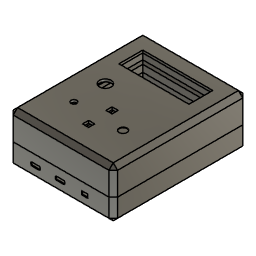
Enclosure (Autodesk Fusion 360 design; units mm, degrees)
Autodesk Fusion 360 part; units mm, degrees
sketch "Sketch1" plane through (0, 0, 0) normal (0, 0, 1) x (1, 0, 0)
  line L0 (0, 0) -> (100, 0)
  line L1 (100, 0) -> (100, -130)
  line L2 (100, -130) -> (0, -130)
  line L3 (0, -130) -> (0, 0)
  line L4 (-3, -133) -> (-3, 3)
  line L5 (-3, 3) -> (103, 3)
  line L6 (103, 3) -> (103, -133)
  line L7 (103, -133) -> (-3, -133)
  dimension "d1" = 100
  dimension "d2" = 130
  dimension "d3" = -3
  constraint horizontal L0
  constraint vertical L1
  constraint horizontal L2
  constraint vertical L3
  constraint coincident L0.start L3.end
  measures "d1" distance of L0.start L0.end
  measures "d2" distance of L0.start L2.end
extrude "Extrude1" add sketch "Sketch1" against normal blind 3 contours L0 L1 L2 L3 | L4 L5 L6 L7 makes body 1
extrude "Extrude2" add sketch "Sketch1" along normal blind 20 separate body makes body 2
extrude "Extrude5" add 1 faces at (-2, -43.3333, 20) along direction (0, 0, 1) blind 25 separate body on bodies 2 makes body 3
sketch "Sketch2" plane through (0, 0, 45) normal (0, 0, 1) x (-1, 0, 0)
  line L0 (-100, 130) -> (0, 130)
  line L1 (0, 130) -> (0, 0)
  line L2 (0, 0) -> (-100, 0)
  line L3 (-100, 0) -> (-100, 130)
  line L4 (-102, 132) -> (-102, -2)
  line L5 (-102, -2) -> (2, -2)
  line L6 (2, -2) -> (2, 132)
  line L7 (2, 132) -> (-102, 132)
  line L8 (2, -2) -> (-102, -2)
  line L9 (-102, -2) -> (-102, 132)
  line L10 (-102, 132) -> (2, 132)
  line L11 (2, 132) -> (2, -2)
  line L12 (0, 0) -> (-100, 0)
  line L13 (-100, 0) -> (-100, 130)
  line L14 (-100, 130) -> (0, 130)
  line L15 (0, 130) -> (0, 0)
  line L16 (0, 0) -> (-14.45, 0)
  line L17 (-14.45, 0) -> (-14.45, 14.45)
  line L18 (-14.45, 14.45) -> (0, 14.45)
  line L19 (0, 14.45) -> (0, 0)
  line L20 (-14.45, 14.45) -> (-85.55, 14.45)
  line L21 (-85.55, 14.45) -> (-85.55, 38.65)
  line L22 (-85.55, 38.65) -> (-14.45, 38.65)
  line L23 (-14.45, 38.65) -> (-14.45, 14.45)
  line L24 (-85.55, 14.45) -> (-100, 14.45)
  circle A0 centre (-25, 95) radius 2.9
  circle A1 centre (-25, 63) radius 5.95
  line L25 (-48.8, 103.8) -> (-55, 103.8)
  line L26 (-55, 103.8) -> (-55, 110)
  line L27 (-55, 110) -> (-48.8, 110)
  line L28 (-48.8, 110) -> (-48.8, 103.8)
  line L29 (-48.8, 80) -> (-55, 80)
  line L30 (-55, 80) -> (-55, 86.2)
  line L31 (-55, 86.2) -> (-48.8, 86.2)
  line L32 (-48.8, 86.2) -> (-48.8, 80)
  circle A2 centre (-75, 95) radius 4
  line L33 (-100, 130) -> (-75, 130)
  line L34 (-75, 130) -> (-75, 95)
  line L35 (-75, 95) -> (-100, 95)
  line L36 (-100, 95) -> (-100, 130)
  line L37 (-55, 110) -> (-100, 110)
  line L38 (-100, 110) -> (-100, 130)
  line L39 (-100, 130) -> (-55, 130)
  line L40 (-55, 130) -> (-55, 110)
  line L41 (-75, 95) -> (-25, 95)
  line L42 (-25, 95) -> (-25, 63)
  line L43 (-25, 63) -> (-25, 65.0002)
  line L44 (-48.8, 86.2) -> (-48.8, 95)
  line L45 (-48.8, 95) -> (-48.8, 103.8)
  line L46 (-100, 130) -> (0, 130)
  line L47 (0, 130) -> (0, 0)
  line L48 (0, 0) -> (-100, 0)
  line L49 (-100, 0) -> (-100, 130)
  line L50 (-103, 133) -> (-103, -3)
  line L51 (-103, -3) -> (3, -3)
  line L52 (3, -3) -> (3, 133)
  line L53 (3, 133) -> (-103, 133)
  dimension "d8" = 71.1
  dimension "d9" = 24.2
  dimension "d11" = 5.8
  dimension "d12" = 11.9
  dimension "d15" = 6.2
  dimension "d16" = 8
  dimension "d17" = 25
  dimension "d19" = 45
  dimension "d20" = 20
  dimension "d22" = 50
  dimension "d23" = 32
  dimension "d27" = 35
  constraint horizontal L8
  constraint vertical L9
  constraint horizontal L10
  constraint vertical L11
  constraint coincident L4.start L7.end
  constraint coincident L5.end L6.start
  constraint horizontal L12
  constraint vertical L13
  constraint horizontal L14
  constraint vertical L15
  constraint coincident L0.start L3.end
  constraint coincident L1.end L2.start
  constraint horizontal L16
  constraint vertical L17
  constraint horizontal L18
  constraint vertical L19
  constraint horizontal L20
  constraint vertical L21
  constraint horizontal L22
  constraint vertical L23
  constraint coincident L13 L24.end
  constraint perpendicular L13 L24
  constraint equal L18 L24
  constraint equal L17 L18
  constraint horizontal L25
  constraint vertical L26
  constraint horizontal L27
  constraint vertical L28
  constraint horizontal L29
  constraint vertical L30
  constraint horizontal L31
  constraint vertical L32
  constraint equal L25 L26
  constraint equal L26 L32
  constraint equal L29 L32
  constraint horizontal L33
  constraint vertical L34
  constraint horizontal L35
  constraint vertical L36
  constraint coincident A2.centre L34.end
  constraint horizontal L37
  constraint vertical L38
  constraint horizontal L39
  constraint vertical L40
  constraint perpendicular L34 L41
  constraint coincident A0.centre L41.end
  constraint perpendicular L41 L42
  constraint coincident A1.centre L42.end
  constraint parallel L42 L43
  constraint coincident L41 L44.end
  constraint perpendicular L41 L44
  constraint perpendicular L25 L45
  constraint equal L44 L45
  measures "d8" distance of L17.end L20.end
  measures "d9" distance of L17.end L22.end
  measures "d11" diameter of A0
  measures "d12" diameter of A1
  measures "d15" distance of L25.start L25.end
  measures "d16" diameter of A2
  measures "d17" distance of A2.centre L35.end
  measures "d19" distance of L26.end L37.end
  measures "d20" distance of L26.end L39.end
  measures "d22" distance of A2.centre A0.centre
  measures "d23" distance of A0.centre A1.centre
  measures "d27" distance of L14 L41
extrude "Extrude3" add sketch "Sketch2" along normal blind 3 separate body contours L0 L3 L13 L14 L33 L34 L36 L37 L38 L39 L46 L49 | L0 L14 L34 L37 L39 L40 L46 | L3 L13 A2 L34 L35 L36 L37 L49 | L0 L1 L3 L13 L14 L15 L18 L21 L22 L23 L24 L27 L28 A2 L35 L40 L41 L45 L46 L47 L49 | L25 L26 A2 L34 L37 L41 L45 | L2 L3 L12 L13 L17 L20 L24 L48 L49 | L1 L2 L12 L15 L16 L17 L18 L19 L47 L48 | L4 L5 L6 L7 L8 L9 L10 L11 | L50 L51 L52 L53 makes body 4
sketch "Sketch6" plane through (0, 0, 45) normal (0, 0, -1) x (1, 0, 0)
  line L0 (48.8, 86.2) -> (55, 86.2)
  line L1 (55, 86.2) -> (55, 80)
  line L2 (55, 80) -> (48.8, 80)
  line L3 (48.8, 80) -> (48.8, 86.2)
  line L4 (14.45, 38.65) -> (85.55, 38.65)
  line L5 (85.55, 38.65) -> (85.55, 14.45)
  line L6 (85.55, 14.45) -> (14.45, 14.45)
  line L7 (14.45, 14.45) -> (14.45, 38.65)
  circle A0 centre (25, 95) radius 2.9
  circle A1 centre (25, 63) radius 5.95
  circle A2 centre (75, 95) radius 4
  line L8 (48.8, 110) -> (55, 110)
  line L9 (55, 110) -> (55, 103.8)
  line L10 (55, 103.8) -> (48.8, 103.8)
  line L11 (48.8, 103.8) -> (48.8, 110)
  line L12 (103, 133) -> (-3, 133)
  line L13 (-3, 133) -> (-3, -3)
  line L14 (-3, -3) -> (103, -3)
  line L15 (103, -3) -> (103, 133)
  line L16 (5, 5) -> (95, 5)
  line L17 (95, 5) -> (95, 125)
  line L18 (95, 125) -> (5, 125)
  line L19 (5, 125) -> (5, 5)
  line L20 (5, 5) -> (95, 125) construction
  line L21 (95, 5) -> (5, 125) construction
  line L22 (46.9, 78.1) -> (56.9, 78.1)
  line L23 (56.9, 78.1) -> (56.9, 88.1)
  line L24 (56.9, 88.1) -> (46.9, 88.1)
  line L25 (46.9, 88.1) -> (46.9, 78.1)
  line L26 (46.9, 78.1) -> (56.9, 88.1) construction
  line L27 (56.9, 78.1) -> (46.9, 88.1) construction
  line L28 (46.9, 101.9) -> (56.9, 101.9)
  line L29 (56.9, 101.9) -> (56.9, 111.9)
  line L30 (56.9, 111.9) -> (46.9, 111.9)
  line L31 (46.9, 111.9) -> (46.9, 101.9)
  line L32 (46.9, 101.9) -> (56.9, 111.9) construction
  line L33 (56.9, 101.9) -> (46.9, 111.9) construction
  circle A3 centre (25, 95) radius 5
  circle A4 centre (25, 63) radius 10
  line L34 (10, 11.55) -> (90, 11.55)
  line L35 (90, 11.55) -> (90, 41.55)
  line L36 (90, 41.55) -> (10, 41.55)
  line L37 (10, 41.55) -> (10, 11.55)
  line L38 (10, 11.55) -> (90, 41.55) construction
  line L39 (90, 11.55) -> (10, 41.55) construction
  point P0 (50, 65)
  point P1 (51.9, 83.1)
  point P2 (51.9, 106.9)
  point P3 (50, 26.55)
  dimension "d68" = 90
  dimension "d69" = 120
  dimension "d70" = 10
  dimension "d71" = 10
  dimension "d72" = 10
  dimension "d73" = 10
  dimension "d74" = 10
  dimension "d75" = 20
  dimension "d76" = 80
  dimension "d77" = 30
  constraint horizontal L16
  constraint perpendicular L16 L17
  constraint parallel L16 L18
  constraint parallel L17 L19
  constraint coincident L20 P0
  constraint coincident L21 P0
  constraint horizontal L22
  constraint perpendicular L22 L23
  constraint parallel L22 L24
  constraint parallel L23 L25
  constraint coincident L26 P1
  constraint coincident L27 P1
  constraint horizontal L28
  constraint perpendicular L28 L29
  constraint parallel L28 L30
  constraint parallel L29 L31
  constraint coincident L32 P2
  constraint coincident L33 P2
  constraint concentric A0 A3
  constraint concentric A1 A4
  constraint horizontal L34
  constraint perpendicular L34 L35
  constraint parallel L34 L36
  constraint parallel L35 L37
  constraint coincident L38 P3
  constraint coincident L39 P3
  measures "d68" distance of L17.end L18.end
  measures "d69" distance of L16.end L17.end
  measures "d70" distance of L23.end L24.end
  measures "d71" distance of L22.end L23.end
  measures "d72" distance of L29.end L30.end
  measures "d73" distance of L28.end L29.end
  measures "d74" diameter of A3
  measures "d75" diameter of A4
  measures "d76" distance of L35.end L36.end
  measures "d77" distance of L34.end L35.end
extrude "Extrude10" cut sketch "Sketch6" against normal blind 2 contours A2 | L16 L17 L18 L19 bodies 4
chamfer "Chamfer1" distance 0.5 angle 45 15 edges at (55, -83.1, 45) (51.9, -86.2, 45) (48.8, -83.1, 45) (51.9, -80, 45) (51.9, -103.8, 45) (55, -106.9, 45) (51.9, -110, 45) (48.8, -106.9, 45) (27.7037, -96.0487, 45) (50, -38.65, 45) (85.55, -26.55, 45) (50, -14.45, 45) (14.45, -26.55, 45) (30.5473, -65.1516, 45) (78.7293, -96.4465, 47) on bodies 4
sketch "Sketch3" plane through (0, -133, 0) normal (0, -1, 0) x (1, 0, 0)
  line L0 (-3, 0) -> (103, 0)
  line L1 (103, 0) -> (103, 20)
  line L2 (103, 20) -> (-3, 20)
  line L3 (-3, 20) -> (-3, 0)
  line L4 (49, 0) -> (49, 10)
  line L5 (49, 10) -> (24, 10)
  line L6 (28.75, 8.25) -> (19.25, 8.25)
  line L7 (19.25, 8.25) -> (19.25, 11.75)
  line L8 (19.25, 11.75) -> (28.75, 11.75)
  line L9 (28.75, 11.75) -> (28.75, 8.25)
  line L10 (28.75, 8.25) -> (19.25, 11.75) construction
  line L11 (19.25, 8.25) -> (28.75, 11.75) construction
  line L12 (49, 10) -> (56.2134, 10)
  line L13 (44, 10) -> (74, 10)
  line L14 (77.1, 8.15) -> (70.9, 8.15)
  line L15 (70.9, 8.15) -> (70.9, 11.85)
  line L16 (70.9, 11.85) -> (77.1, 11.85)
  line L17 (77.1, 11.85) -> (77.1, 8.15)
  line L18 (77.1, 8.15) -> (70.9, 11.85) construction
  line L19 (70.9, 8.15) -> (77.1, 11.85) construction
  line L20 (53.75, 11.75) -> (44.25, 11.75)
  line L21 (44.25, 11.75) -> (44.25, 8.25)
  line L22 (44.25, 8.25) -> (53.75, 8.25)
  line L23 (53.75, 8.25) -> (53.75, 11.75)
  line L24 (53.75, 11.75) -> (44.25, 8.25) construction
  line L25 (44.25, 11.75) -> (53.75, 8.25) construction
  point P0 (24, 10)
  point P1 (74, 10)
  point P2 (49, 10)
  dimension "d30" = 10
  dimension "d31" = 9.5
  dimension "d32" = 3.5
  dimension "d35" = 25
  dimension "d39" = 6.2
  dimension "d40" = 3.7
  dimension "d43" = 52
  dimension "d45" = 9.5
  dimension "d46" = 3.5
  dimension "d47" = 25
  constraint perpendicular L0 L4
  constraint perpendicular L4 L5
  constraint horizontal L6
  constraint perpendicular L6 L7
  constraint parallel L6 L8
  constraint parallel L7 L9
  constraint coincident L10 P0
  constraint coincident L11 P0
  constraint coincident P0 L5.end
  constraint perpendicular L4 L12
  constraint coincident L0 L4.start
  constraint parallel L12 L13
  constraint horizontal L14
  constraint perpendicular L14 L15
  constraint parallel L14 L16
  constraint parallel L15 L17
  constraint coincident L18 P1
  constraint coincident L19 P1
  constraint coincident P1 L13.end
  constraint horizontal L20
  constraint perpendicular L20 L21
  constraint parallel L20 L22
  constraint parallel L21 L23
  constraint coincident L24 P2
  constraint coincident L25 P2
  constraint coincident P2 L4.end
  measures "d30" distance of L4.start P2
  measures "d31" distance of L7.end L8.end
  measures "d32" distance of L6.end L7.end
  measures "d35" distance of P2 P0
  measures "d39" distance of L15.end L16.end
  measures "d40" distance of L14.end L15.end
  measures "d43" distance of L3 L4
  measures "d45" distance of L21.end L22.end
  measures "d46" distance of L20.end L21.end
  measures "d47" distance of P1 P2
extrude "Extrude4" cut sketch "Sketch3" against normal blind 3 contours L4 L5 L13 L21 L22 | L4 L12 L13 L22 L23 | L5 L12 L13 L20 L21 L23 | L6 L7 L8 L9 | L14 L15 L16 L17 bodies 2
fillet "Fillet1" radius 1 8 edges at (53.75, -131.5, 8.25) (44.25, -131.5, 8.25) (44.25, -131.5, 11.75) (53.75, -131.5, 11.75) (28.75, -131.5, 11.75) (28.75, -131.5, 8.25) (19.25, -131.5, 8.25) (19.25, -131.5, 11.75) on bodies 2
combine "Combine1" operation add target body 1 tool bodies 2
combine "Combine2" operation add target body 4 tool bodies 3
sketch "Sketch4" plane through (0, -130, 0) normal (0, 1, 0) x (-1, 0, 0)
  line L0 (-19.25, 10.75) -> (-19.25, 9.25)
  arc A0 (-20.25, 8.25) -> (-19.25, 9.25) centre (-20.25, 9.25) ccw
  line L1 (-20.25, 8.25) -> (-27.75, 8.25)
  arc A1 (-28.75, 9.25) -> (-27.75, 8.25) centre (-27.75, 9.25) ccw
  line L2 (-28.75, 9.25) -> (-28.75, 10.75)
  arc A2 (-27.75, 11.75) -> (-28.75, 10.75) centre (-27.75, 10.75) ccw
  line L3 (-27.75, 11.75) -> (-20.25, 11.75)
  arc A3 (-19.25, 10.75) -> (-20.25, 11.75) centre (-20.25, 10.75) ccw
  line L4 (-52.75, 11.75) -> (-45.25, 11.75)
  arc A4 (-44.25, 10.75) -> (-45.25, 11.75) centre (-45.25, 10.75) ccw
  line L5 (-44.25, 10.75) -> (-44.25, 9.25)
  arc A5 (-45.25, 8.25) -> (-44.25, 9.25) centre (-45.25, 9.25) ccw
  line L6 (-45.25, 8.25) -> (-52.75, 8.25)
  arc A6 (-53.75, 9.25) -> (-52.75, 8.25) centre (-52.75, 9.25) ccw
  line L7 (-53.75, 9.25) -> (-53.75, 10.75)
  arc A7 (-52.75, 11.75) -> (-53.75, 10.75) centre (-52.75, 10.75) ccw
  line L8 (-70.9, 11.85) -> (-70.9, 8.15)
  line L9 (-70.9, 8.15) -> (-77.1, 8.15)
  line L10 (-77.1, 8.15) -> (-77.1, 11.85)
  line L11 (-77.1, 11.85) -> (-70.9, 11.85)
  line L12 (-100, 0) -> (0, 0)
  line L13 (0, 0) -> (0, 20)
  line L14 (0, 20) -> (-100, 20)
  line L15 (-100, 20) -> (-100, 0)
  line L16 (-9, 4) -> (-89, 4)
  line L17 (-89, 4) -> (-89, 16)
  line L18 (-89, 16) -> (-9, 16)
  line L19 (-9, 16) -> (-9, 4)
  line L20 (-9, 4) -> (-89, 16) construction
  line L21 (-89, 4) -> (-9, 16) construction
  point P0 (-49, 10)
  dimension "d56" = 80
  dimension "d57" = 12
  constraint horizontal L16
  constraint perpendicular L16 L17
  constraint parallel L16 L18
  constraint parallel L17 L19
  constraint coincident L20 P0
  constraint coincident L21 P0
  measures "d56" distance of L17.end L18.end
  measures "d57" distance of L16.end L17.end
extrude "Extrude7" cut sketch "Sketch4" against normal blind 2 contours L16 L17 L18 L19 bodies 1
chamfer "Chamfer3" distance 2 angle 45 8 edges at (49, -132, 4) (9, -132, 10) (89, -131, 16) (89, -132, 10) (49, -132, 16) (89, -131, 4) (9, -131, 4) (9, -131, 16) on bodies 1
sketch "Sketch5" plane through (0, 0, 20) normal (0, 0, -1) x (1, 0, 0)
  line L0 (103, 133) -> (-3, 133)
  line L1 (-3, 133) -> (-3, -3)
  line L2 (-3, -3) -> (103, -3)
  line L3 (103, -3) -> (103, 133)
  line L4 (0, 130) -> (100, 130)
  line L5 (100, 130) -> (100, 0)
  line L6 (100, 0) -> (0, 0)
  line L7 (0, 0) -> (0, 130)
  line L8 (99.75, 129.75) -> (99.75, 0.25)
  line L9 (99.75, 0.25) -> (0.25, 0.25)
  line L10 (0.25, 0.25) -> (0.25, 129.75)
  line L11 (0.25, 129.75) -> (99.75, 129.75)
  line L12 (98, 128) -> (98, 2)
  line L13 (98, 2) -> (2, 2)
  line L14 (2, 2) -> (2, 128)
  line L15 (2, 128) -> (98, 128)
  dimension "d61" = 0.25
  dimension "d62" = 2
extrude "Extrude8" add sketch "Sketch5" against normal blind 3 contours L4 L5 L6 L7 | L8 L9 L10 L11 bodies 4
chamfer "Chamfer4" distance 2 angle 45 4 edges at (50, 0, 23) (0, -65, 23) (100, -65, 23) (50, -130, 23) on bodies 4
extrude "Extrude9" add sketch "Sketch5" along normal blind 4 contours L8 L9 L10 L11 bodies 4
chamfer "Chamfer2" distance 4.4 angle 45 16 edges at (-3, -65, 48) (50, 3, 48) (103, -65, 48) (103, 3, 34) (103, -133, 34) (-3, -133, 34) (-3, 3, 34) (50, -133, 48) (103, 3, 8.5) (103, -65, -3) (103, -133, 8.5) (50, -133, -3) (-3, -133, 8.5) (50, 3, -3) (-3, 3, 8.5) (-3, -65, -3) on bodies 1 4
sketch "Sketch7" plane through (0, 0, 0) normal (0, 0, 1) x (-1, 0, 0)
  line L0 (-100, 130) -> (-100, 0)
  line L1 (-100, 0) -> (0, 0)
  line L2 (0, 0) -> (0, 130)
  line L3 (0, 130) -> (-100, 130)
  line L4 (-97, 3) -> (-3, 3)
  line L5 (-3, 3) -> (-3, 127)
  line L6 (-3, 127) -> (-97, 127)
  line L7 (-97, 127) -> (-97, 3)
  line L8 (-97, 3) -> (-3, 127) construction
  line L9 (-3, 3) -> (-97, 127) construction
  point P0 (-50, 65)
  dimension "d82" = 94
  dimension "d83" = 124
  constraint horizontal L4
  constraint perpendicular L4 L5
  constraint parallel L4 L6
  constraint parallel L5 L7
  constraint coincident L8 P0
  constraint coincident L9 P0
  measures "d82" distance of L5.end L6.end
  measures "d83" distance of L4.end L5.end
extrude "Extrude12" cut sketch "Sketch7" against normal blind 2 contours L4 L5 L6 L7 bodies 1
equation "d43 = ( 104 / 2 ) * 1 mm"
